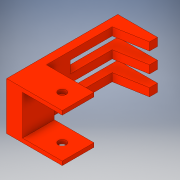
# Autodesk Inventor part: claw
Saved by Autodesk Inventor 2019 (Build 230136000, 136)
## iProperties
Created: 2019-03-05
Part Number: claw
Material: 일반
Document SubType Name: Modeling
Designer: Jeong Ji Hoon
Density: 1 g/cm^3
Appearance: 기본값
Author: Jeong Ji Hoon
Autodesk Inventor part; units mm, degrees
ref_plane "YZ Plane" through (0, 0, 0) normal (1, 0, 0) x (0, 1, 0)
ref_plane "XZ Plane" through (0, 0, 0) normal (0, 1, 0) x (-1, 0, 0)
ref_plane "XY Plane" through (0, 0, 0) normal (0, 0, 1) x (1, 0, 0)
sketch "스케치1" plane through (0, 0, 0) normal (0, 1, 0) x (-1, 0, 0)
  line L0 (0, 0) -> (70, 0)
  line L1 (70, 0) -> (70, -140)
  line L2 (70, -140) -> (20, -140)
  line L3 (20, -140) -> (20, -130)
  line L4 (20, -130) -> (60, -122.9469)
  line L5 (60, -122.9469) -> (60, -40)
  line L6 (60, -40) -> (0, -40)
  line L7 (0, -40) -> (0, 0)
  dimension "d0" = 60
  dimension "d1" = 40
  dimension "d2" = 140
  dimension "d3" = 50
  dimension "d4" = 100
  dimension "d5" = 10
  dimension "d6" = 70
  constraints: 16 end point, 5 perpendicular, 1 horizontal, 1 parallel
  measures "d0" distance of L5.end L6.end
  measures "d1" distance of L6.end L0.start
  measures "d2" distance of L0.end L1.end
  measures "d3" distance of L1.end L2.end
  measures "d4" angle of L3 L4
  measures "d5" distance of L2.end L3.end
  measures "d6" distance between parallel lines of L7 L1
extrude "돌출1" add sketch "스케치1" along normal blind 60
sketch "스케치2" plane through (0, 0, 0) normal (1, 0, 0) x (0, 0, -1)
  line L0 (40, 0) -> (0, 0) projected
  line L1 (40, 0) -> (40, 60) projected
  line L2 (0, 60) -> (40, 60) projected
  line L3 (0, 0) -> (0, 60) projected
  line L4 (40, 0) -> (40, 60) projected
  line L5 (0, 5) -> (40, 5)
  line L6 (40, 5) -> (40, 55)
  line L7 (40, 55) -> (0, 55)
  line L8 (0, 55) -> (0, 5)
  dimension "d9" = 5
  dimension "d10" = 5
  constraints: 8 end point, 2 parallel, 2 point on line, 1 horizontal, 1 perpendicular
  measures "d9" distance between parallel lines of L2 L7
  measures "d10" distance between parallel lines of L0 L5
extrude "돌출2" cut sketch "스케치2" against normal blind 50 contours L5 L3 L7 L1
sketch "스케치3" plane through (-20, 0, -130) normal (1, 0, 0) x (0, 0, -1)
  line L0 (10, 0) -> (0, 0) projected
  line L1 (10, 0) -> (10, 60) projected
  line L2 (0, 60) -> (10, 60) projected
  line L3 (0, 0) -> (0, 60) projected
  line L4 (10, 35) -> (-60, 35)
  line L5 (-60, 35) -> (-60, 50)
  line L6 (-60, 50) -> (10, 50)
  line L7 (10, 50) -> (10, 35)
  line L8 (10, 0) -> (10, 60) projected
  line L9 (10, 10) -> (-60, 10)
  line L10 (-60, 10) -> (-60, 25)
  line L11 (-60, 25) -> (10, 25)
  line L12 (10, 25) -> (10, 10)
  line L13 (-90, 60) -> (-7.0531, 60) projected
  line L14 (-7.0531, 0) -> (-90, 0) projected
  point P0 (-130, 0)
  dimension "d13" = 70
  dimension "d14" = 15
  dimension "d15" = 70
  dimension "d16" = 15
  dimension "d17" = 10
  dimension "d18" = 10
  constraints: 16 end point, 4 parallel, 2 horizontal, 2 perpendicular, 2 point on line
  measures "d13" distance of L5.end L6.end
  measures "d14" distance of L4.end L5.end
  measures "d15" distance of L10.end L11.end
  measures "d16" distance of L9.end L10.end
  measures "d17" distance between parallel lines of L13 L6
  measures "d18" distance between parallel lines of L14 L9
extrude "돌출3" cut sketch "스케치3" against normal blind 50 contours L9 L3 L11 L1 | L9 L10 L11 L3 | L4 L3 L6 L1 | L4 L5 L6 L3
sketch "스케치4" plane through (0, 60, 0) normal (0, 1, 0) x (1, 0, 0)
  line L0 (-70, 0) -> (0, 0) projected
  line L1 (0, 0) -> (0, 40) projected
  point P0 (-20, 20)
  dimension "d21" = 20
  dimension "d22" = 20
  measures "d21" distance from line of L0 point (-20, 20)
  measures "d22" distance from line of L1 point (-20, 20)
hole "구멍1" at (-20, 60, -20) direction (0, -1, 0) diameter 10 end through all
